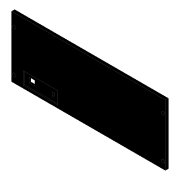
# Autodesk Inventor part: Electronics Housing Back Pannel
Saved by Autodesk Inventor 2020 (Build 240168000, 168)
## iProperties
Created: 2021-08-28
Part Number: Electronics Housing Back Pannel
Material: Generic
Document SubType Name: Modeling
Designer: Coy
Density: 1 g/cm^3
Appearance: Anodized - Black
Author: Coy
Autodesk Inventor part; units mm, degrees
ref_plane "YZ Plane" through (0, 0, 0) normal (1, 0, 0) x (0, 1, 0)
ref_plane "XZ Plane" through (0, 0, 0) normal (0, 1, 0) x (-1, 0, 0)
ref_plane "XY Plane" through (0, 0, 0) normal (0, 0, 1) x (1, 0, 0)
sketch "Sketch1" plane through (0, 0, 0) normal (0, 0, 1) x (1, 0, 0)
  line L0 (-10, 1.25) -> (-5, 1.25) construction
  line L1 (-10, 1.25) -> (-10, 0) construction
  line L2 (0, 0) -> (-10, 0) construction
  line L3 (0, 0) -> (0, 131) construction
  line L4 (0, 131) -> (-320, 131) construction
  line L5 (-320, 119.0545) -> (-320, 131) construction
  line L6 (-320, 119.0545) -> (-10, 119.0545) construction
  line L7 (-10, 119.0545) -> (-10, 10.75) construction
  line L8 (-5, 10.75) -> (-10, 10.75) construction
  line L9 (-5, 10.75) -> (-5, 1.25) construction
  circle A0 centre (-5, 104.0545) radius 3 construction
  circle A1 centre (-5, 15) radius 3 construction
  line L10 (-165, 119.0545) -> (-165, 0) construction
  circle A2 centre (-325, 104.0545) radius 3 construction
  circle A3 centre (-325, 15) radius 3 construction
  line L11 (0, 0) -> (-330, 0)
  line L12 (-330, 0) -> (-330, 131)
  line L13 (-330, 131) -> (0, 131)
  line L14 (0, 131) -> (0, 0)
  circle A4 centre (-325, 104.0545) radius 2.25
  circle A5 centre (-325, 15) radius 2.25
  circle A6 centre (-5, 15) radius 2.25
  circle A7 centre (-5, 104.0545) radius 2.25
  point P0 (0, 3)
  dimension "d0" = 330
  dimension "d1" = 4.5
  dimension "d2" = 4.5
  dimension "d3" = 4.5
  dimension "d4" = 4.5
  constraints: 30 end point, 8 centre point, 6 horizontal, 6 vertical, 4 coincident, 2 parallel, 2 symmetric about line, 1 midpoint, 1 perpendicular, 1 point on line, 18 other
  measures "d0" distance of L12.end L13.end
  measures "d1" diameter of A4
  measures "d2" diameter of A5
  measures "d3" diameter of A7
  measures "d4" diameter of A6
extrude "Extrusion1" add sketch "Sketch1" along normal blind 6.5
sketch "Sketch2" plane through (0, 0, 6.5) normal (0, 0, 1) x (1, 0, 0)
  circle A0 centre (-325, 104.0545) radius 2.25 projected
  circle A1 centre (-325, 15) radius 2.25 projected
  circle A2 centre (-5, 15) radius 2.25 projected
  circle A3 centre (-5, 104.0545) radius 2.25 projected
  circle A4 centre (-325, 104.0545) radius 2.25 projected
  circle A5 centre (-325, 104.0545) radius 3.55
  circle A6 centre (-325, 15) radius 2.25 projected
  circle A7 centre (-325, 15) radius 3.55
  circle A8 centre (-5, 15) radius 2.25 projected
  circle A9 centre (-5, 15) radius 3.55
  circle A10 centre (-5, 104.0545) radius 2.25 projected
  circle A11 centre (-5, 104.0545) radius 3.55
  point P0 (0, 0)
  dimension "d7" = 7.1
  dimension "d8" = 7.1
  dimension "d9" = 7.1
  dimension "d10" = 7.1
  constraints: 4 centre point, 4 coincident
  measures "d7" diameter of A5
  measures "d8" diameter of A7
  measures "d9" diameter of A11
  measures "d10" diameter of A9
extrude "Extrusion2" cut sketch "Sketch2" against normal blind 4.5
sketch "Sketch3" plane through (0, 0, 6.5) normal (0, 0, 1) x (1, 0, 0)
  line L0 (95.8094, 14.15) -> (-425.3856, 14.15) construction
  line L1 (-330, 0) -> (0, 0) construction
  line L2 (-282.73, 175.8186) -> (-282.73, -97.3031) construction
  line L3 (0, 0) -> (0, 131) construction
  line L4 (-294.3061, 24.8296) -> (-283.1861, 24.8296)
  arc A0 (-282.73, 24.31) -> (-283.1861, 24.8296) centre (-283.1861, 24.3696) ccw
  arc A1 (-294.3061, 24.8296) -> (-294.7622, 24.31) centre (-294.3061, 24.3696) ccw
  line L5 (-294.7622, 24.31) -> (-294.7622, 14.15)
  line L6 (-294.7622, 14.15) -> (-282.73, 14.15)
  line L7 (-282.73, 14.15) -> (-282.73, 24.31)
  line L8 (-262.63, 24.65) -> (-262.63, 14.15) construction
  line L9 (-262.63, 14.15) -> (-262.63, 24.65) construction
  arc A2 (-262.1302, 25.1657) -> (-262.63, 24.65) centre (-262.1302, 24.6657) ccw construction
  arc A3 (-262.1302, 25.1657) -> (-262.63, 24.65) centre (-262.1302, 24.6657) ccw construction
  line L10 (-262.1302, 25.1657) -> (-254.1302, 25.1657) construction
  line L11 (-262.1302, 25.1657) -> (-254.1302, 25.1657) construction
  arc A4 (-253.6267, 24.7049) -> (-254.1302, 25.1657) centre (-254.1252, 24.6658) ccw construction
  arc A5 (-253.6267, 24.7049) -> (-254.1302, 25.1657) centre (-254.1252, 24.6658) ccw construction
  line L12 (-253.6267, 14.15) -> (-253.6267, 24.7049) construction
  line L13 (-262.63, 14.15) -> (-253.6267, 14.15) construction
  line L14 (-282.73, 14.15) -> (-262.63, 14.15) construction
  line L15 (-283.1861, 25.0296) -> (-294.3061, 25.0296)
  arc A6 (-294.3061, 25.0296) -> (-294.9622, 24.2982) centre (-294.3061, 24.3696) ccw
  line L16 (-294.9622, 24.2982) -> (-294.9622, 13.95)
  line L17 (-294.9622, 13.95) -> (-282.53, 13.95)
  line L18 (-282.53, 13.95) -> (-282.53, 24.2982)
  arc A7 (-282.53, 24.2982) -> (-283.1861, 25.0296) centre (-283.1861, 24.3696) ccw
  line L19 (-253.6267, 14.15) -> (-262.6267, 14.15) construction
  line L20 (-262.6267, 14.15) -> (-262.6267, 24.65) construction
  line L21 (-262.1267, 25.15) -> (-254.1267, 25.15) construction
  line L22 (-253.6267, 24.65) -> (-253.6267, 14.15) construction
  arc A8 (-262.1267, 25.15) -> (-262.6267, 24.65) centre (-262.1267, 24.65) ccw construction
  arc A9 (-253.6267, 24.65) -> (-254.1267, 25.15) centre (-254.1267, 24.65) ccw construction
  line L23 (-262.8267, 24.65) -> (-262.8267, 13.95) construction
  line L24 (-262.8267, 13.95) -> (-253.4267, 13.95) construction
  line L25 (-253.4267, 13.95) -> (-253.4267, 24.65) construction
  arc A10 (-253.4267, 24.65) -> (-254.1267, 25.35) centre (-254.1267, 24.65) ccw construction
  line L26 (-254.1267, 25.35) -> (-262.1267, 25.35) construction
  arc A11 (-262.1267, 25.35) -> (-262.8267, 24.65) centre (-262.1267, 24.65) ccw construction
  line L27 (-245.6267, 14.15) -> (-241.1267, 14.15)
  line L28 (-241.1267, 14.15) -> (-241.1267, 21.9)
  line L29 (-241.1267, 21.9) -> (-245.6267, 21.9)
  line L30 (-245.6267, 21.9) -> (-245.6267, 14.15)
  point P0 (-262.6267, 25.15)
  point P1 (-253.6267, 25.15)
  dimension "d13" = 14.15
  dimension "d14" = 282.73
  dimension "d36" = 20.1
  dimension "d37" = 10.16
  dimension "d38" = 10.16
  dimension "d39" = 12.0322
  dimension "d40" = 11.12
  dimension "d41" = 10.5
  dimension "d44" = 8
  dimension "d45" = 0.46
  dimension "d46" = 0.46
  dimension "d47" = 0.5
  dimension "d48" = 0.5
  dimension "d51" = 9.0033
  dimension "d52" = 0.5
  dimension "d53" = 0.5
  dimension "d54" = 0.4985
  dimension "d55" = 0.4997
  dimension "d57" = 0
  dimension "d58" = 0
  dimension "d59" = 0.2
  dimension "d60" = 9
  dimension "d61" = 11
  dimension "d62" = 0.5
  dimension "d63" = 0.2
  dimension "d64" = 4.5
  dimension "d65" = 7.75
  dimension "d66" = 8
  constraints: 58 end point, 24 point on circle, 12 centre point, 10 perpendicular, 6 horizontal, 6 parallel, 6 tangent, 5 point on line, 1 collinear, 1 equal radius, 1 vertical, 10 other
  measures "d13" distance between parallel lines of L1 L0
  measures "d14" distance between parallel lines of L3 L2
  measures "d36" distance between parallel lines of L8 L7
  measures "d37" distance of L6.end L7.end
  measures "d38" distance of L5.start L5.end
  measures "d39" distance of L5.end L6.end
  measures "d40" distance of L4.start L4.end
  measures "d41" distance of L8.start L8.end
  measures "d44" distance of L10.start L10.end
  measures "d45" radius of A0
  measures "d46" radius of A1
  measures "d47" radius of A2
  measures "d48" radius of A4
  measures "d51" distance between parallel lines of L8 L12
  measures "d52" distance from line of L10 A2.centre
  measures "d53" distance from line of L10 A5.centre
  measures "d54" distance from line of L12 A5.centre
  measures "d55" distance from line of L8 A2.centre
  measures "d57" distance between parallel lines of L2 L7
  measures "d58" distance between parallel lines of L0 L14
  measures "d59" distance between parallel lines of L4 L15
  measures "d60" distance of point (-262.627, 25.15) point (-253.627, 25.15)
  measures "d61" distance of L19.end point (-262.627, 25.15)
  measures "d62" radius of A8
  measures "d63" radial gap between concentric circles of A8 A11
  measures "d64" distance of L29.end L28.end
  measures "d65" distance of L28.end L27.end
  measures "d66" distance between parallel lines of L12 L30
extrude "Extrusion3" cut sketch "Sketch3" against normal through all contours L4 A0 L7 L6 L5 A1 | A7 L18 L17 L16 A6 L15 | L30 L29 L28 L27
sketch "Sketch4" plane through (0, 0, 6.5) normal (0, 0, 1) x (1, 0, 0)
  line L0 (-304.9622, 5.95) -> (-231.1267, 5.95)
  line L1 (-231.1267, 5.95) -> (-231.1267, 33.0296)
  line L2 (-231.1267, 33.0296) -> (-304.9622, 33.0296)
  line L3 (-304.9622, 33.0296) -> (-304.9622, 5.95)
  line L4 (-294.9622, 13.95) -> (-294.9622, 24.2982) projected
  line L5 (-241.1267, 21.9) -> (-241.1267, 14.15) projected
  line L6 (-294.3061, 25.0296) -> (-283.1861, 25.0296) projected
  line L7 (-282.53, 13.95) -> (-294.9622, 13.95) projected
  point P0 (0, 0)
  dimension "d69" = 10
  dimension "d70" = 10
  dimension "d71" = 8
  dimension "d72" = 8
  constraints: 8 end point, 2 parallel, 1 horizontal, 1 perpendicular
  measures "d69" distance between parallel lines of L3 L4
  measures "d70" distance between parallel lines of L5 L1
  measures "d71" distance between parallel lines of L2 L6
  measures "d72" distance between parallel lines of L0 L7
extrude "Extrusion4" cut sketch "Sketch4" against normal blind 2.5
equation "\"d2\" = d1"
equation "\"d3\" = d1"
equation "\"d4\" = d1"
equation "\"d8\" = d7"
equation "\"d9\" = d7"
equation "\"d10\" = d7"
body "Solid1"
